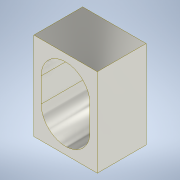
# Autodesk Inventor part: shadeHolder
Saved by Autodesk Inventor 2021.2 (Build 252289000, 289)
## iProperties
Created: 2021-02-12
Part Number: shadeHolder
Material: PC/ABS Plastic
Document SubType Name: Modeling
Designer: robst
Density: 0.357273 g/cm^3
Appearance: Silver
Author: robst
Autodesk Inventor part; units mm, degrees
ref_plane "YZ Plane" through (0, 0, 0) normal (1, 0, 0) x (0, 1, 0)
ref_plane "XZ Plane" through (0, 0, 0) normal (0, 1, 0) x (-1, 0, 0)
ref_plane "XY Plane" through (0, 0, 0) normal (0, 0, 1) x (1, 0, 0)
sketch "Sketch1" plane through (0, 0, 0) normal (0, 0, 1) x (1, 0, 0)
  line L0 (0, -3.175) -> (0, 3.175) construction
  line L1 (6.35, -3.175) -> (6.35, 3.175)
  line L2 (-6.35, 3.175) -> (-6.35, -3.175)
  arc A0 (-6.35, -3.175) -> (6.35, -3.175) centre (0, -3.175) ccw
  arc A1 (6.35, 3.175) -> (-6.35, 3.175) centre (0, 3.175) ccw
  line L3 (-8.255, -11.43) -> (8.255, -11.43)
  line L4 (8.255, -11.43) -> (8.255, 11.43)
  line L5 (8.255, 11.43) -> (-8.255, 11.43)
  line L6 (-8.255, 11.43) -> (-8.255, -11.43)
  line L7 (-8.255, -11.43) -> (8.255, 11.43) construction
  line L8 (8.255, -11.43) -> (-8.255, 11.43) construction
  point P0 (0, 0)
  dimension "d0" = 6.35
  dimension "d1" = 19.05
  dimension "d2" = 1.905
  dimension "d3" = 1.905
  constraints: 20 end point, 4 point on circle, 4 tangent, 3 midpoint, 3 parallel, 2 centre point, 2 perpendicular, 1 vertical
  measures "d0" radius of A1
  measures "d2" distance edge to line of A0 L3
  measures "d3" distance between parallel lines of L4 L1
extrude "Extrusion1" add sketch "Sketch1" along normal mid plane 12.7
body "Solid1"
